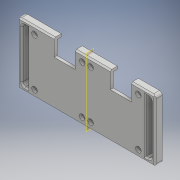
# Autodesk Inventor part: front-stereo2
Saved by Autodesk Inventor 2017 (Build 210142000, 142)
## iProperties
Created: 2017-04-10
Part Number: front-stereo2
Material: Generic
Document SubType Name: Modeling
Designer: Matt Bierner
Density: 1 g/cm^3
Appearance: Default
Author: Matt Bierner
Autodesk Inventor part; units mm, degrees
ref_plane "XZ Plane" through (0, 0, 0) normal (0, 1, 0) x (-1, 0, 0)
ref_plane "XY Plane" through (0, 0, 0) normal (0, 0, 1) x (1, 0, 0)
sketch "Sketch1" plane through (0, 0, 0) normal (0, 1, 0) x (-1, 0, 0)
  line L0 (49, 22) -> (-49, 22)
  line L1 (-49, 22) -> (-49, -22)
  line L2 (-49, -22) -> (49, -22)
  line L3 (49, -22) -> (49, 22)
  line L4 (49, 22) -> (-49, -22) construction
  line L5 (-49, 22) -> (49, -22) construction
  point P0 (0, 0)
  dimension "d0" = 44
  dimension "d1" = 98
  constraints: 12 end point, 2 midpoint, 2 parallel, 1 horizontal, 1 perpendicular
  measures "d0" distance of L2.end L0.start
  measures "d1" distance of L1.end L2.end
extrude "Extrusion1" add sketch "Sketch1" along normal blind 5
sketch "Sketch2" plane through (0, 5, 0) normal (0, 1, 0) x (1, 0, 0)
  line L0 (68.6, 0) -> (-68.6, 0) projected
  line L1 (0, 30.8) -> (0, -30.8) projected
  line L2 (-40, -20) -> (0, -20)
  line L3 (0, -20) -> (0, 20)
  line L4 (0, 20) -> (-40, 20)
  line L5 (-40, 20) -> (-40, -20)
  line L6 (-40, -20) -> (0, 20) construction
  line L7 (0, -20) -> (-40, 20) construction
  point P0 (0, 0)
  point P1 (-20, 0)
  dimension "d4" = 40
  dimension "d5" = 40
  dimension "d6" = 0
  constraints: 12 end point, 2 midpoint, 2 parallel, 1 horizontal, 1 perpendicular, 1 point on line
  measures "d4" distance of L3.end L4.end
  measures "d5" distance of L2.end L3.end
  measures "d6" distance between parallel lines of L1 L3
extrude "Extrusion2" cut sketch "Sketch2" against normal blind 3
sketch "Sketch3" plane through (0, 2, 0) normal (0, 1, 0) x (1, 0, 0)
  line L0 (0, -20) -> (-40, -20) projected
  line L1 (0, 20) -> (0, -20) projected
  line L2 (-40, 20) -> (0, 20) projected
  line L3 (-40, -20) -> (-40, 20) projected
  line L4 (-40, -20) -> (-40, 20) projected
  line L5 (-40, 20) -> (-34, 20)
  line L6 (-34, 20) -> (-34, 14)
  line L7 (-34, 14) -> (-40, 14)
  line L8 (-40, 14) -> (-40, 20)
  line L9 (0, 20) -> (0, -20) projected
  line L10 (0, 20) -> (-6, 20)
  line L11 (-6, 20) -> (-6, 14)
  line L12 (-6, 14) -> (0, 14)
  line L13 (0, 14) -> (0, 20)
  line L14 (0, -20) -> (-40, -20) projected
  line L15 (-40, -20) -> (-34, -20)
  line L16 (-34, -20) -> (-34, -14)
  line L17 (-34, -14) -> (-40, -14)
  line L18 (-40, -14) -> (-40, -20)
  line L19 (0, -20) -> (-6, -20)
  line L20 (-6, -20) -> (-6, -14)
  line L21 (-6, -14) -> (0, -14)
  line L22 (0, -14) -> (0, -20)
  point P0 (0, 0)
  dimension "d9" = 6
  dimension "d10" = 6
  dimension "d11" = 6
  dimension "d12" = 6
  dimension "d13" = 6
  dimension "d14" = 6
  dimension "d15" = 6
  dimension "d69" = 6
  constraints: 32 end point, 8 parallel, 4 horizontal, 4 perpendicular
  measures "d9" distance of L6.end L7.end
  measures "d10" distance of L5.end L6.end
  measures "d11" distance of L12.end L11.end
  measures "d12" distance of L17.end L16.end
  measures "d13" distance of L16.end L15.end
  measures "d14" distance of L20.end L21.end
  measures "d15" distance of L19.end L20.end
  measures "d69" distance of L10.end L11.end
extrude "Extrusion3" add sketch "Sketch3" along normal blind 2 contours L0 L20 L21 L1 | L0 L3 L17 L16 | L12 L11 L2 L1 | L3 L2 L6 L7
sketch "Sketch5" plane through (0, 5, 0) normal (0, 1, 0) x (1, 0, 0)
  line L0 (68.6, 0) -> (-68.6, 0) projected
  line L1 (-42, 19) -> (-46, 19)
  line L2 (-46, 19) -> (-46, -19)
  line L3 (-46, -19) -> (-42, -19)
  line L4 (-42, -19) -> (-42, 19)
  line L5 (-42, 19) -> (-46, -19) construction
  line L6 (-46, 19) -> (-42, -19) construction
  line L7 (-40, -20) -> (-40, 20) projected
  point P0 (0, 0)
  point P1 (-44, 0)
  dimension "d25" = 38
  dimension "d26" = 2
  dimension "d27" = 4
  constraints: 12 end point, 2 midpoint, 2 parallel, 1 horizontal, 1 perpendicular, 1 point on line
  measures "d25" distance of L3.end L1.start
  measures "d26" distance between parallel lines of L7 L4
  measures "d27" distance of L2.end L3.end
extrude "Extrusion5" cut sketch "Sketch5" against normal through all
sketch "Sketch6" plane through (0, 2, 0) normal (0, 1, 0) x (1, 0, 0)
  line L0 (-34, 20) -> (-34, 14) projected
  line L1 (-34, 14) -> (-40, 14) projected
  line L2 (-40, -14) -> (-40, 14) projected
  line L3 (-40, -14) -> (-34, -14) projected
  line L4 (-34, -14) -> (-34, -20) projected
  line L5 (-6, -20) -> (-34, -20) projected
  line L6 (-6, -20) -> (-6, -14) projected
  line L7 (-6, -14) -> (0, -14) projected
  line L8 (0, 14) -> (0, -14) projected
  line L9 (0, 14) -> (-6, 14) projected
  line L10 (-6, 14) -> (-6, 20) projected
  line L11 (-34, 20) -> (-6, 20) projected
  line L12 (-6, -20) -> (-34, -20) projected
  line L13 (-23, -20) -> (-8, -20)
  line L14 (-8, -20) -> (-8, -10)
  line L15 (-8, -10) -> (-23, -10)
  line L16 (-23, -10) -> (-23, -20)
  line L17 (-8, -20) -> (-23, -20)
  line L18 (-23, -20) -> (-23, -30)
  line L19 (-23, -30) -> (-8, -30)
  line L20 (-8, -30) -> (-8, -20)
  point P0 (0, 0)
  dimension "d38" = 10
  dimension "d39" = 15
  dimension "d40" = 8
  dimension "d70" = 10
  constraints: 16 end point, 4 parallel, 2 horizontal, 2 perpendicular, 1 point on line
  measures "d38" distance of L15.end L13.start
  measures "d39" distance of L14.end L15.end
  measures "d40" distance between parallel lines of L8 L14
  measures "d70" distance of L18.end L17.end
extrude "Extrusion6" cut sketch "Sketch6" along normal through all both and the other way through all contours L16 L15 L14 L5 | L5 L20 L19 L18
pattern_linear "Rectangular Pattern1" count 2 spacing 40 along (1, 0, 0) of "Extrusion2", "Extrusion3", "Extrusion6"
mirror "Mirror2" about plane through (0, 0, 0) normal (1, 0, 0) of "Extrusion5"
chamfer "Chamfer3" distance 1 angle 45 6 edges at (-49, 0, 0) (0, 0, -22) (40.5, 0, 22) (4.5, 0, 22) (-36, 0, 22) (49, 0, 0)
fillet "Fillet4" radius 2 2 edges at (-46, 2.5, -19) (-46, 2.5, 19)
fillet "Fillet5" radius 2 4 edges at (-49, 3, -22) (-49, 3, 22) (49, 3, 22) (49, 3, -22)
fillet "Fillet6" radius 2 2 edges at (46, 2.5, 19) (46, 2.5, -19)
chamfer "Chamfer4" distance 1 angle 45 12 edges at (-42, 0, 0) (-43, 0, 19) (-45.4142, 0, 18.4142) (-46, 0, 0) (-45.4142, 0, -18.4142) (-43, 0, -19) (46, 0, 0) (45.4142, 0, -18.4142) (43, 0, -19) (45.4142, 0, 18.4142) (43, 0, 19) (42, 0, 0)
sketch "Sketch8" plane through (0, 0, 0) normal (0, -1, 0) x (1, 0, 0)
  line L0 (0, 30.8) -> (0, -30.8) projected
  line L1 (-68.6, 0) -> (68.6, 0) projected
  line L2 (37, 17) -> (3, 17)
  line L3 (3, 17) -> (3, -17)
  line L4 (3, -17) -> (37, -17)
  line L5 (37, -17) -> (37, 17)
  line L6 (37, 17) -> (3, -17) construction
  line L7 (3, 17) -> (37, -17) construction
  point P0 (0, 0)
  point P1 (20, 0)
  dimension "d59" = 34
  dimension "d60" = 34
  dimension "d61" = 20
  constraints: 12 end point, 2 midpoint, 2 parallel, 1 horizontal, 1 perpendicular, 1 point on line
  measures "d59" distance of L4.end L3.end
  measures "d60" distance of L2.end L3.end
  measures "d61" distance from line of L0 point (20, 0)
hole "Hole1" at (37, 0, -17) at (37, 0, 17) at (3, 0, 17) at (3, 0, -17) direction (0, 1, 0) diameter 2 depth 12 tip angle 118 counterbore diameter 4 counterbore depth 2
mirror "Mirror3" about plane through (0, 0, 0) normal (1, 0, 0) of "Hole1"
body "Solid1"
